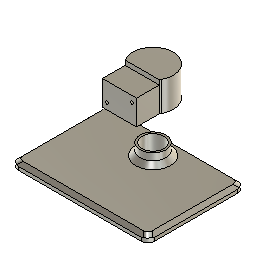
Monitor Mount for LG 22MK430H-B (Autodesk Fusion 360 design; units mm, degrees)
Autodesk Fusion 360 part; units mm, degrees
sketch "Sketch1" plane through (0, 0, 0) normal (0, 1, 0) x (1, 0, 0) in component "Rough draft"
  line L0 (15, -11) -> (-15, -11)
  line L1 (-15, -11) -> (-15, 11)
  line L2 (-15, 11) -> (15, 11)
  line L3 (15, 11) -> (15, -11)
  line L4 (15, -11) -> (-15, 11) construction
  line L5 (-15, -11) -> (15, 11) construction
  line L6 (11, 5.5) -> (-11, 5.5) construction
  line L7 (-11, 5.5) -> (-11, -5.5) construction
  line L8 (-11, -5.5) -> (11, -5.5) construction
  line L9 (11, -5.5) -> (11, 5.5) construction
  line L10 (11, 5.5) -> (-11, -5.5) construction
  line L11 (-11, 5.5) -> (11, -5.5) construction
  circle A0 centre (11, -5.5) radius 1.25
  circle A1 centre (-11, 5.5) radius 1.25
  dimension "d1" = 22
  dimension "d2" = 30
  dimension "d3" = 22
  dimension "d4" = 11
  dimension "d5" = 2.5
  constraint horizontal L0
  constraint perpendicular L0 L1
  constraint parallel L0 L2
  constraint parallel L1 L3
  constraint coincident L4 origin
  constraint coincident L5 origin
  constraint horizontal L6
  constraint perpendicular L6 L7
  constraint parallel L6 L8
  constraint parallel L7 L9
  constraint coincident L10 origin
  constraint coincident L11 origin
  constraint coincident L8.end L9.start
  constraint coincident L6.end L7.start
  constraint equal A0 A1
  measures "d1" distance of L0.end L1.end
  measures "d2" distance of L1.end L2.end
  measures "d3" distance of L7.end L8.end
  measures "d4" distance of L6.end L7.end
  measures "d5" diameter of A0
extrude "Extrude1" add sketch "Sketch1" along normal blind 20 contours L0 L1 L2 L3 | A0 | A1 makes body 1 in component "Rough draft"
sketch "Sketch2" plane through (0, 0, 11) normal (0, 0, 1) x (-1, 0, 0) in component "Rough draft"
  line L0 (15, 0) -> (-15, 0)
  line L1 (-15, 0) -> (-15, -20)
  line L2 (-15, -20) -> (15, -20)
  line L3 (15, -20) -> (15, 0)
  line L4 (0, 0) -> (0, -29.525) construction
  circle A0 centre (0, -29.525) radius 9.525
  arc A1 (-15.6683, -21.2681) -> (15.6683, -21.2681) centre (0, -29.525) ccw
  line L5 (-15, -20) -> (-15.6683, -21.2681)
  line L6 (15, -20) -> (15.6683, -21.2681)
  dimension "d8" = 19.05
  dimension "d9" = 8.1858
  constraint coincident L4.start origin
  constraint perpendicular L0 L4
  constraint coincident L4.end A0.centre
  constraint tangent L2 A0
  constraint coincident L1.end L2.start
  constraint coincident L2.end L3.start
  constraint tangent A1 L5
  constraint tangent A1 L6
  measures "d8" diameter of A0
  measures "d9" distance of A0 A1
extrude "Extrude2" add sketch "Sketch2" against normal blind 22 contours L2 A1 L5 L6 bodies 1 in component "Rough draft"
extrude "Extrude3" add sketch "Sketch2" along normal blind 4 contours A0 | L2 A1 L5 L6 bodies 1 in component "Rough draft"
extrude "Extrude4" add sketch "Sketch2" against normal blind 0.1 contours A0 bodies 1 in component "Rough draft"
chamfer "Chamfer1" distance 1 angle 45 1 edges at (8.8804, 32.9694, 10.9) on bodies 1 in component "Rough draft"
extrude "Extrude5" cut sketch "Sketch1" along normal blind 10 contours A0 | A1 bodies 1 in component "Rough draft"
sketch "Sketch3" plane through (0, 0, 0) normal (0, 1, 0) x (1, 0, 0) in component "Rough draft"
  circle A0 centre (-11, 5.5) radius 1.25
  circle A1 centre (11, -5.5) radius 1.25
  line L0 (-11, 5.5) -> (-11, 3.7322) construction
  line L1 (-11, 4.25) -> (-10.4822, 4.25)
  line L2 (-10.4822, 4.25) -> (-10.1161, 4.6161)
  line L3 (-11, 4.25) -> (-11.5178, 4.25)
  line L4 (-11.5178, 4.25) -> (-11.8839, 4.6161)
  line L5 (11, -5.5) -> (11, -6.75) construction
  line L6 (11, -6.75) -> (11.5178, -6.75)
  line L7 (11.5178, -6.75) -> (11.8839, -6.3839)
  line L8 (11, -6.75) -> (10.4822, -6.75)
  line L9 (10.4822, -6.75) -> (10.1161, -6.3839)
  dimension "d20" = 135
  dimension "d21" = 135
  constraint coincident A0.centre L0.start
  constraint vertical L0
  constraint coincident A0 L1.start
  constraint coincident L0 L1.start
  constraint tangent A0 L1
  constraint coincident A0 L2.end
  constraint tangent A0 L2
  constraint symmetric L0 L1.start L3.start
  constraint symmetric L0 L1.end L3.end
  constraint symmetric L0 L2.end L4.end
  constraint coincident A1.centre L5.start
  constraint coincident A1 L5.end
  constraint vertical L5
  constraint tangent A1 L6
  constraint coincident A1 L7.end
  constraint tangent A1 L7
  constraint symmetric L6.start L5 L8.start
  constraint symmetric L5 L6.end L8.end
  constraint symmetric L5 L7.end L9.end
  measures "d20" angle of L1 L2
  measures "d21" angle of L6 L7
extrude "Extrude6" cut sketch "Sketch3" along normal blind 10 contours A0 L3 L4 | A0 L1 L2 | A1 L8 L9 | A1 L6 L7 bodies 1 in component "Rough draft"
ref_plane "WorkPlane1" through (0, 26.1998, -61) normal (0, 0, -1) x (-1, 0, 0) in component "Rough draft"
sketch "Base" plane through (0, 0, -61) normal (0, 0, -1) x (-1, 0, 0) in component "Rough draft"
  circle A0 centre (0, 29.525) radius 9.525
  line L0 (60, -35) -> (-60, -35)
  line L1 (-60, -35) -> (-60, 50)
  line L2 (-60, 50) -> (60, 50)
  line L3 (60, 50) -> (60, -35)
  line L4 (0, 50) -> (0, -35) construction
  line L5 (0, 20) -> (6.5325, 20) construction
  circle A1 centre (0, 29.525) radius 11.325
  dimension "d25" = 55
  dimension "d26" = 30
  dimension "d27" = 120
  dimension "d32" = 1.8
  constraint horizontal L0
  constraint vertical L1
  constraint horizontal L2
  constraint vertical L3
  constraint midpoint L2 L4.start
  constraint midpoint L0 L4.end
  constraint coincident A0.centre L4
  constraint coincident L4 L5.start
  constraint coincident A0 L5.start
  constraint tangent A0 L5
  constraint concentric A0 A1
  measures "d25" distance of L0 L5.start
  measures "d26" distance of L2 L5.start
  measures "d27" distance of L1.end L2.end
  measures "d32" distance of A0 A1
extrude "Extrude7" add sketch "Base" against normal blind 1 separate body contours A0 makes body 2 in component "Rough draft"
extrude "Extrude9" add sketch "Base" against normal blind 16 contours A1 bodies 2 in component "Rough draft"
extrude "Extrude8" add sketch "Base" against normal blind 6 contours L0 L1 L2 L3 bodies 2 in component "Rough draft"
chamfer "Chamfer2" distance 3 angle 45 4 edges at (0, -35, -55) (-60, 7.5, -55) (0, 50, -55) (60, 7.5, -55) on bodies 2 in component "Rough draft"
fillet "Fillet1" radius 6 8 edges at (60, -35, -59.5) (58.5, -33.5, -56.5) (58.5, 48.5, -56.5) (60, 50, -59.5) (-60, -35, -59.5) (-58.5, -33.5, -56.5) (-60, 50, -59.5) (-58.5, 48.5, -56.5) on bodies 2 in component "Rough draft"
chamfer "Chamfer3" distance 4 angle 45 1 edges at (10.5586, 33.6203, -55) on bodies 2 in component "Rough draft"
component "Rough draft" placed x (1, 0, 0) y (0, 1, 0) z (0, 0, 1) at (0, 0, 0)
named bodies: "Monitor Mount", "Base"
